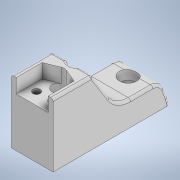
# Autodesk Inventor part: Part2
Saved by Autodesk Inventor 2020.3 (Build 243373000, 373)
## iProperties
Created: 2021-03-28
Part Number: Part2
Material: Generic
Document SubType Name: Modeling
Designer: sanyi
Density: 1 g/cm^3
Appearance: Default
Author: sanyi
Autodesk Inventor part; units mm, degrees
ref_plane "YZ Plane" through (0, 0, 0) normal (1, 0, 0) x (0, 1, 0)
ref_plane "XZ Plane" through (0, 0, 0) normal (0, 1, 0) x (-1, 0, 0)
sketch "Sketch1" plane through (0, 0, 0) normal (0, 1, 0) x (-1, 0, 0)
  line L0 (8.5, 19) -> (-8.5, 19)
  line L1 (-8.5, 19) -> (-8.5, -28)
  line L2 (-8.5, -28) -> (8.5, -28)
  line L3 (8.5, -28) -> (8.5, 19)
  line L4 (35.537, 0) -> (-37.6285, 0) construction
  line L5 (0, 76.31) -> (0, -83.8259) construction
  circle A0 centre (0, -20) radius 2.05
  circle A1 centre (0, 0) radius 2.05
  line L6 (6.5, 19) -> (6.5, 12.5)
  line L7 (6.5, 12.5) -> (-6.5, 12.5)
  line L8 (-6.5, 12.5) -> (-6.5, 19)
  line L9 (5.2605, 14) -> (-5.0586, 14)
  circle A2 centre (-3.25, 14) radius 1.5
  circle A3 centre (3.25, 14) radius 1.5
  line L10 (6.5, 12.5) -> (6.5, 8.5)
  line L11 (6.5, 8.5) -> (-6.5, 8.5)
  line L12 (-6.5, 8.5) -> (-6.5, 12.5)
  circle A4 centre (0, 8.5) radius 2.5
  line L13 (6.5, 8.5) -> (0.9615, 6.1923)
  line L14 (-0.9615, 6.1923) -> (-6.5, 8.5)
  dimension "d0" = 17
  dimension "d1" = 20
  dimension "d2" = 4.1
  dimension "d3" = 8
  dimension "d4" = 19
  dimension "d7" = 13
  dimension "d8" = 6.5
  dimension "d9" = 3
  dimension "d11" = 1.5
  dimension "d12" = 6.5
  dimension "d13" = 4
  dimension "d14" = 5
  constraints: 30 end point, 9 point on line, 7 parallel, 5 centre point, 2 equal radius, 2 horizontal, 2 perpendicular, 2 point on circle, 2 tangent, 1 collinear, 1 midpoint, 1 symmetric about line, 1 vertical, 2 other
  measures "d0" distance of L1.end L2.end
  measures "d1" distance of A0.centre point (0, 0)
  measures "d2" diameter of A1
  measures "d3" distance from line of L2 A0.centre
  measures "d4" distance from line of L0 point (0, 0)
  measures "d7" distance of L6.end L7.end
  measures "d8" distance of L6.start L6.end
  measures "d9" diameter of A2
  measures "d11" distance between parallel lines of L7 L9
  measures "d12" distance of A2.centre A3.centre
  measures "d13" distance between parallel lines of L7 L11
  measures "d14" diameter of A4
extrude "Extrusion1" add sketch "Sketch1" along normal blind 20 contours L6 L7 A3 L9 A2 L8 L0 | L10 L11 A4 L12 L7 | L7 A2 L9 A3 | A3 L9 | L13 A4 L11 | A2 L9 | L11 A4 L14 | A3 L9 | A2 L9
extrude "Extrusion2" add sketch "Sketch1" along normal blind 25.8 contours L3 L2 L1 L0 L8 L12 L14 A4 L13 L10 L6
sketch "Sketch3" plane through (0, 20, 0) normal (0, 1, 0) x (1, 0, 0)
  circle A0 centre (3.25, -14) radius 1.5 projected
  circle A1 centre (-3.25, -14) radius 1.5 projected
  point P0 (0, 0)
extrude "Extrusion4" cut sketch "Sketch3" against normal blind 4.3
sketch "Sketch5" plane through (0, 25.8, 0) normal (0, 1, 0) x (1, 0, 0)
  circle A0 centre (0, 0) radius 2.05 projected
  circle A1 centre (0, 20) radius 2.05 projected
  circle A2 centre (0, 0) radius 3.5
  circle A3 centre (0, 20) radius 3.5
  dimension "d29" = 7
  dimension "d30" = 7
  constraints: 2 centre point, 2 coincident
  measures "d29" diameter of A2
  measures "d30" diameter of A3
extrude "Extrusion6" cut sketch "Sketch5" against normal blind 19.8
sketch "Sketch6" plane through (0, 25.8, 0) normal (0, 1, 0) x (1, 0, 0)
  circle A0 centre (0, 0) radius 3.5 projected
  circle A1 centre (0, 20) radius 3.5 projected
  circle A2 centre (0, 20) radius 3.5 projected
  circle A3 centre (0, 0) radius 3.5 projected
  line L0 (-8.5, -19) -> (-6.5, -19) projected
  line L1 (-6.5, -19) -> (-6.5, -8.5) projected
  line L2 (-6.5, -8.5) -> (-0.9615, -6.1923) projected
  arc A4 (0.9615, -6.1923) -> (-0.9615, -6.1923) centre (0, -8.5) ccw projected
  line L3 (0.9615, -6.1923) -> (6.5, -8.5) projected
  line L4 (6.5, -8.5) -> (6.5, -19) projected
  line L5 (6.5, -19) -> (8.5, -19) projected
  line L6 (8.5, -19) -> (8.5, 28) projected
  line L7 (8.5, 28) -> (-8.5, 28) projected
  line L8 (-8.5, 28) -> (-8.5, -19) projected
  line L9 (-8.5, 28) -> (-8.5, -19) projected
  line L10 (-8.5, 7) -> (8.5, 7)
  dimension "d41" = 13
  constraints: 2 end point, 2 point on line, 1 coincident, 1 perpendicular
  measures "d41" distance from line of A1.centre L10
extrude "Extrusion7" cut sketch "Sketch6" against normal blind 15.8 contours L8 L7 L6 L10
chamfer "Chamfer2" distance 10 distance2 15.8 1 edges at (0, 25.8, -7)
chamfer "Chamfer3" distance 8 distance2 3 1 edges at (0, 10, -28) measured on face at (0, 9.5, -28)
fillet "Fillet1" radius 5 2 edges at (0, 10, -25) (0, 2, -28)
fillet "Fillet1" radius 10 1 edges at (0, 10, -7)
fillet "Fillet2" radius 1 3 edges at (5.1514, 25.8, 3) (0, 25.8, 3.5) (-5.1514, 25.8, 3)
fillet "Fillet3" radius 1 18 edges at (8.5, 11.2399, -7.6826) (8.5, 19.9934, -0.6751) (8.5, 25.676, 3.0683) (8.5, 25.8, 11.2753) (8.5, 9.1096, -24.383) (8.5, 4.8023, -26.9491) (8.5, 1.9855, -27.9198) (8.5, 0.5467, -28) (8.5, 10, -17.0202) (-8.5, 9.1096, -24.383) (-8.5, 4.8023, -26.9491) (-8.5, 1.9855, -27.9198) (-8.5, 0.5467, -28) (-8.5, 11.2399, -7.6826) (-8.5, 19.9934, -0.6751) (-8.5, 25.676, 3.0683) (-8.5, 25.8, 11.2753) (-8.5, 10, -17.0202)
ref_plane "Work Plane1" through (-6.5, 0, 8.5) normal (0, -0.4226183, 0.9063078) x (1, 0, 0)
sketch "Sketch7" plane through (-6.5, 0, 8.5) normal (0, -0.4226183, 0.9063078) x (1, 0, 0)
  circle A0 centre (6.5, 1) radius 2.5
  line L0 (0, 0) -> (13, 0) projected
  line L1 (6.5, -2.449) -> (6.5, 4.9828)
  line L2 (9, -4.085) -> (4, -4.085)
  line L3 (4, -4.085) -> (4, 1)
  line L4 (4, 1) -> (9, 1)
  line L5 (9, 1) -> (9, -4.085)
  point P0 (6.5, -3.5923)
  point P1 (6.5, 0)
  point P2 (6.5, 0)
  dimension "d47" = 5
  dimension "d50" = 1
  constraints: 10 end point, 2 parallel, 2 perpendicular, 2 point on circle, 2 point on line, 1 centre point, 1 horizontal, 1 midpoint, 1 tangent
  measures "d47" diameter of A0
  measures "d50" distance of point (6.5, 0) A0.centre
extrude "Extrusion8" cut sketch "Sketch7" along normal blind 10
fillet "Fillet4" radius 2 1 edges at (0, 2.6961, 11)
body "Solid1"
